dadheadphonesv1 (Autodesk Fusion 360 design; units mm, degrees)
Autodesk Fusion 360 part; units mm, degrees
sketch "Sketch1" plane through (0, 0, 0) normal (0, 1, 0) x (1, 0, 0)
  line L0 (0, 0) -> (25, 0)
  line L1 (25, 0) -> (25, -8)
  line L2 (25, -8) -> (-36, -8)
  line L3 (-36, -8) -> (-36, -21)
  line L4 (-36, -21) -> (-44, -21)
  line L5 (-44, -21) -> (-44, 0)
  line L6 (-44, 0) -> (-6, 0)
  line L7 (-6, 0) -> (-6, 28)
  line L8 (-6, 28) -> (40, 28)
  line L9 (40, 28) -> (40, 20)
  line L10 (40, 20) -> (0, 20)
  line L11 (0, 20) -> (0, 0)
  line L12 (-6, 28) -> (-25.6058, 0)
  line L13 (-6, 19.2828) -> (-19.5019, 0)
  dimension "d1" = 20
  dimension "d2" = 8
  dimension "d3" = 8
  dimension "d4" = 40
  dimension "d5" = 25
  dimension "d6" = 6
  dimension "d8" = 36
  dimension "d9" = 8
  dimension "d10" = 13
  dimension "d12" = 8
  dimension "d15" = 5
  dimension "d16" = 35
  constraint coincident L0.start L11.end
  constraint horizontal L0
  constraint perpendicular L0 L1
  constraint perpendicular L1 L2
  constraint perpendicular L2 L3
  constraint perpendicular L1 L4
  constraint perpendicular L4 L5
  constraint perpendicular L5 L6
  constraint perpendicular L6 L7
  constraint perpendicular L5 L8
  constraint perpendicular L8 L9
  constraint perpendicular L9 L10
  constraint perpendicular L0 L11
  constraint coincident L6 L12.end
  constraint coincident L7 L13.start
  constraint coincident L6 L13.end
  constraint parallel L12 L13
  measures "d1" distance of L0 L10
  measures "d2" distance of L8.end L9.end
  measures "d3" distance of L0.end L1.end
  measures "d4" distance of L9.end L10.end
  measures "d5" distance of L0.start L0.end
  measures "d6" distance of L7 L11
  measures "d8" distance of L3 L11
  measures "d9" distance of L3.end L4.end
  measures "d10" distance of L2 L4
  measures "d12" distance of L2 L6
  measures "d15" distance of L12 L13
  measures "d16" angle of L7 L12
extrude "Extrude1" add sketch "Sketch1" along normal blind 15 contours L0 L1 L2 L3 L4 L5 L6 L7 L8 L9 L10 L11 | L6 L7 L12 L13
